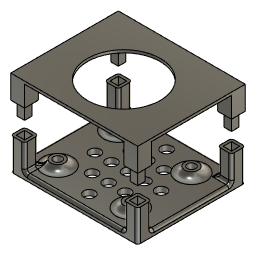
Joystick+Holder+Rev+3 (Autodesk Fusion 360 design; units mm, degrees)
Autodesk Fusion 360 part; units mm, degrees
sketch "Joystick Layout" plane through (0, 0, 0) normal (0, 0, 1) x (1, 0, 0)
  line L0 (15.6333, 7.2313) -> (49.6333, 7.2313)
  line L1 (49.6333, 7.2313) -> (49.6333, 34.2313)
  line L2 (49.6333, 34.2313) -> (15.6333, 34.2313)
  line L3 (15.6333, 34.2313) -> (15.6333, 7.2313)
  line L4 (23.1333, 10.7313) -> (39.1333, 10.7313)
  line L5 (39.1333, 10.7313) -> (39.1333, 26.7313)
  line L6 (39.1333, 26.7313) -> (23.1333, 26.7313)
  line L7 (23.1333, 26.7313) -> (23.1333, 10.7313)
  line L8 (26.1333, 10.7313) -> (36.1333, 10.7313)
  line L9 (36.1333, 10.7313) -> (36.1333, 8.2313)
  line L10 (36.1333, 8.2313) -> (26.1333, 8.2313)
  line L11 (26.1333, 8.2313) -> (26.1333, 10.7313)
  line L12 (23.1333, 13.7313) -> (20.6333, 13.7313)
  line L13 (20.6333, 13.7313) -> (20.6333, 23.7313)
  line L14 (20.6333, 23.7313) -> (23.1333, 23.7313)
  line L15 (23.1333, 23.7313) -> (23.1333, 13.7313)
  circle A0 centre (32.1333, 19.7313) radius 6
  circle A1 centre (32.1333, 19.7313) radius 2
  line L16 (30.681, 21.1063) -> (30.681, 18.3562)
  line L17 (33.681, 20.998) -> (33.681, 18.4645)
  circle A2 centre (18.1333, 9.7313) radius 1.5
  circle A3 centre (18.1333, 31.7313) radius 1.5
  circle A4 centre (44.6333, 31.7313) radius 1.5
  circle A5 centre (44.6333, 9.7313) radius 1.5
  circle A6 centre (32.1333, 19.7313) radius 13
  line L18 (9.6333, 40.2313) -> (55.6333, 40.2313)
  line L19 (55.6333, 40.2313) -> (55.6333, 1.2313)
  line L20 (55.6333, 1.2313) -> (9.6333, 1.2313)
  line L21 (9.6333, 1.2313) -> (9.6333, 40.2313)
  line L22 (9.6333, 40.2313) -> (14.6333, 40.2313)
  line L23 (14.6333, 40.2313) -> (14.6333, 35.2313)
  line L24 (14.6333, 35.2313) -> (9.6333, 35.2313)
  line L25 (9.6333, 35.2313) -> (9.6333, 40.2313)
  line L26 (55.6333, 40.2313) -> (50.6333, 40.2313)
  line L27 (50.6333, 40.2313) -> (50.6333, 35.2313)
  line L28 (50.6333, 35.2313) -> (55.6333, 35.2313)
  line L29 (55.6333, 35.2313) -> (55.6333, 40.2313)
  line L30 (9.6333, 1.2313) -> (14.6333, 1.2313)
  line L31 (14.6333, 1.2313) -> (14.6333, 6.2313)
  line L32 (14.6333, 6.2313) -> (9.6333, 6.2313)
  line L33 (9.6333, 6.2313) -> (9.6333, 1.2313)
  line L34 (55.6333, 1.2313) -> (50.6333, 1.2313)
  line L35 (50.6333, 1.2313) -> (50.6333, 6.2313)
  line L36 (50.6333, 6.2313) -> (55.6333, 6.2313)
  line L37 (55.6333, 6.2313) -> (55.6333, 1.2313)
  line L38 (10.6333, 39.2313) -> (13.6333, 39.2313)
  line L39 (13.6333, 39.2313) -> (13.6333, 36.2313)
  line L40 (13.6333, 36.2313) -> (10.6333, 36.2313)
  line L41 (10.6333, 36.2313) -> (10.6333, 39.2313)
  line L42 (51.6333, 39.2313) -> (54.6333, 39.2313)
  line L43 (54.6333, 39.2313) -> (54.6333, 36.2313)
  line L44 (54.6333, 36.2313) -> (51.6333, 36.2313)
  line L45 (51.6333, 36.2313) -> (51.6333, 39.2313)
  line L46 (51.6333, 5.2313) -> (54.6333, 5.2313)
  line L47 (54.6333, 5.2313) -> (54.6333, 2.2313)
  line L48 (54.6333, 2.2313) -> (51.6333, 2.2313)
  line L49 (51.6333, 2.2313) -> (51.6333, 5.2313)
  line L50 (10.6333, 5.2313) -> (13.6333, 5.2313)
  line L51 (13.6333, 5.2313) -> (13.6333, 2.2313)
  line L52 (13.6333, 2.2313) -> (10.6333, 2.2313)
  line L53 (10.6333, 2.2313) -> (10.6333, 5.2313)
  circle A7 centre (18.1333, 31.7313) radius 2.5
  circle A8 centre (44.6333, 31.7313) radius 2.5
  circle A9 centre (44.6333, 9.7313) radius 2.5
  circle A10 centre (18.1333, 9.7313) radius 2.5
  circle A11 centre (32.1333, 19.7313) radius 13.2
  line L54 (10.7833, 39.0813) -> (13.4833, 39.0813)
  line L55 (13.4833, 39.0813) -> (13.4833, 36.3813)
  line L56 (13.4833, 36.3813) -> (10.7833, 36.3813)
  line L57 (10.7833, 36.3813) -> (10.7833, 39.0813)
  line L58 (51.7833, 39.0813) -> (54.4833, 39.0813)
  line L59 (54.4833, 39.0813) -> (54.4833, 36.3813)
  line L60 (54.4833, 36.3813) -> (51.7833, 36.3813)
  line L61 (51.7833, 36.3813) -> (51.7833, 39.0813)
  line L62 (54.4833, 2.3813) -> (51.7833, 2.3813)
  line L63 (51.7833, 2.3813) -> (51.7833, 5.0813)
  line L64 (51.7833, 5.0813) -> (54.4833, 5.0813)
  line L65 (54.4833, 5.0813) -> (54.4833, 2.3813)
  line L66 (10.7833, 5.0813) -> (13.4833, 5.0813)
  line L67 (13.4833, 5.0813) -> (13.4833, 2.3813)
  line L68 (13.4833, 2.3813) -> (10.7833, 2.3813)
  line L69 (10.7833, 2.3813) -> (10.7833, 5.0813)
  dimension "d1" = 34
  dimension "d2" = 27
  dimension "d3" = 16
  dimension "d4" = 16
  dimension "d5" = 10
  dimension "d6" = 2.5
  dimension "d7" = 2.5
  dimension "d8" = 10
  dimension "d9" = 3
  dimension "d10" = 3
  dimension "d11" = 1
  dimension "d12" = 12
  dimension "d13" = 9
  dimension "d14" = 9
  dimension "d15" = 4
  dimension "d16" = 3
  dimension "d17" = 5
  dimension "d18" = 3
  dimension "d19" = 3
  dimension "d20" = 2.5
  dimension "d21" = 2.5
  dimension "d22" = 2.5
  dimension "d23" = 2.5
  dimension "d24" = 3
  dimension "d25" = 3
  dimension "d26" = 2.5
  dimension "d27" = 2.5
  dimension "d28" = 26.5
  dimension "d29" = 26.5
  dimension "d30" = 26
  dimension "d31" = 5
  dimension "d32" = 5
  dimension "d33" = 5
  dimension "d34" = 5
  dimension "d35" = 1
  dimension "d36" = 1
  dimension "d37" = 1
  dimension "d38" = 5
  dimension "d39" = 5
  dimension "d40" = 5
  dimension "d41" = 5
  dimension "d42" = 1
  dimension "d43" = 3
  dimension "d44" = 3
  dimension "d45" = 1
  dimension "d46" = 1
  dimension "d47" = 3
  dimension "d48" = 3
  dimension "d49" = 1
  dimension "d50" = 1
  dimension "d51" = 3
  dimension "d52" = 3
  dimension "d53" = 1
  dimension "d54" = 1
  dimension "d55" = 3
  dimension "d56" = 3
  dimension "d57" = 1
  dimension "d58" = 1
  dimension "d59" = 5
  dimension "d60" = 5
  dimension "d61" = 5
  dimension "d62" = 5
  dimension "d100" = 26.4
  dimension "d107" = 2.7
  dimension "d108" = 2.7
  dimension "d109" = 0.15
  dimension "d110" = 0.15
  dimension "d111" = 2.7
  dimension "d112" = 2.7
  dimension "d113" = 0.15
  dimension "d114" = 0.15
  dimension "d115" = 2.7
  dimension "d116" = 2.7
  dimension "d117" = 0.15
  dimension "d118" = 0.15
  dimension "d119" = 2.7
  dimension "d120" = 2.7
  dimension "d121" = 0.15
  dimension "d122" = 0.15
  constraint horizontal L0
  constraint vertical L1
  constraint horizontal L2
  constraint vertical L3
  constraint horizontal L4
  constraint vertical L5
  constraint horizontal L6
  constraint vertical L7
  constraint horizontal L8
  constraint vertical L9
  constraint horizontal L10
  constraint vertical L11
  constraint coincident L4 L8.start
  constraint horizontal L12
  constraint vertical L13
  constraint horizontal L14
  constraint vertical L15
  constraint coincident L7 L12.start
  constraint concentric A0 A1
  constraint coincident A1 L16.start
  constraint coincident A1 L16.end
  constraint vertical L16
  constraint coincident A1 L17.start
  constraint coincident A1 L17.end
  constraint parallel L16 L17
  constraint concentric A0 A6
  constraint horizontal L18
  constraint vertical L19
  constraint horizontal L20
  constraint vertical L21
  constraint horizontal L22
  constraint vertical L23
  constraint horizontal L24
  constraint vertical L25
  constraint horizontal L26
  constraint vertical L27
  constraint horizontal L28
  constraint vertical L29
  constraint horizontal L30
  constraint vertical L31
  constraint horizontal L32
  constraint vertical L33
  constraint horizontal L34
  constraint vertical L35
  constraint horizontal L36
  constraint vertical L37
  constraint horizontal L38
  constraint vertical L39
  constraint horizontal L40
  constraint vertical L41
  constraint horizontal L42
  constraint vertical L43
  constraint horizontal L44
  constraint vertical L45
  constraint horizontal L46
  constraint vertical L47
  constraint horizontal L48
  constraint vertical L49
  constraint horizontal L50
  constraint vertical L51
  constraint horizontal L52
  constraint vertical L53
  constraint concentric A3 A7
  constraint concentric A4 A8
  constraint concentric A5 A9
  constraint concentric A2 A10
  constraint concentric A1 A11
  constraint horizontal L54
  constraint vertical L55
  constraint horizontal L56
  constraint vertical L57
  constraint horizontal L58
  constraint vertical L59
  constraint horizontal L60
  constraint vertical L61
  constraint horizontal L62
  constraint vertical L63
  constraint horizontal L64
  constraint vertical L65
  constraint horizontal L66
  constraint vertical L67
  constraint horizontal L68
  constraint vertical L69
  measures "d1" distance of L0.start L0.end
  measures "d2" distance of L0.start L2.end
  measures "d3" distance of L4.start L4.end
  measures "d4" distance of L4.start L6.end
  measures "d5" distance of L8.start L8.end
  measures "d6" distance of L8.start L10.end
  measures "d7" distance of L12.start L12.end
  measures "d8" distance of L12.start L14.end
  measures "d9" distance of L4 L12
  measures "d10" distance of L7 L11
  measures "d11" distance of L0 L10
  measures "d12" diameter of A0
  measures "d13" distance of L8 A0.centre
  measures "d14" distance of L7 A0.centre
  measures "d15" diameter of A1
  measures "d16" distance of L16 L17
  measures "d17" distance of L3 L13
  measures "d18" diameter of A2
  measures "d19" diameter of A3
  measures "d20" distance of L3 A3.centre
  measures "d21" distance of L2 A3.centre
  measures "d22" distance of L3 A2.centre
  measures "d23" distance of L0 A2.centre
  measures "d24" diameter of A4
  measures "d25" diameter of A5
  measures "d26" distance of L0 A5.centre
  measures "d27" distance of L2 A4.centre
  measures "d28" distance of A3.centre A4.centre
  measures "d29" distance of A2.centre A5.centre
  measures "d30" diameter of A6
  measures "d31" distance of L18.start L22.end
  measures "d32" distance of L18.start L24.end
  measures "d33" distance of L18.end L26.end
  measures "d34" distance of L18.end L28.end
  measures "d35" distance of L3 L23
  measures "d36" distance of L2 L24
  measures "d37" distance of L1 L27
  measures "d38" distance of L20.end L30.end
  measures "d39" distance of L19.end L34.end
  measures "d40" distance of L19.end L36.end
  measures "d41" distance of L20.end L32.end
  measures "d42" distance of L0 L32
  measures "d43" distance of L38.start L38.end
  measures "d44" distance of L38.start L40.end
  measures "d45" distance of L18 L38
  measures "d46" distance of L25 L41
  measures "d47" distance of L42.start L42.end
  measures "d48" distance of L42.start L44.end
  measures "d49" distance of L19 L43
  measures "d50" distance of L18 L42
  measures "d51" distance of L46.start L46.end
  measures "d52" distance of L46.start L48.end
  measures "d53" distance of L36 L46
  measures "d54" distance of L37 L47
  measures "d55" distance of L50.start L50.end
  measures "d56" distance of L50.start L52.end
  measures "d57" distance of L32 L50
  measures "d58" distance of L31 L51
  measures "d59" diameter of A7
  measures "d60" diameter of A8
  measures "d61" diameter of A9
  measures "d62" diameter of A10
  measures "d100" diameter of A11
  measures "d107" distance of L54.start L54.end
  measures "d108" distance of L54.start L56.end
  measures "d109" distance of L38 L54
  measures "d110" distance of L41 L57
  measures "d111" distance of L58.start L58.end
  measures "d112" distance of L58.start L60.end
  measures "d113" distance of L42 L58
  measures "d114" distance of L45 L61
  measures "d115" distance of L62.start L62.end
  measures "d116" distance of L62.start L64.end
  measures "d117" distance of L46 L64
  measures "d118" distance of L49 L63
  measures "d119" distance of L66.start L66.end
  measures "d120" distance of L66.start L68.end
  measures "d121" distance of L50 L66
  measures "d122" distance of L53 L69
extrude "Extrude1" add sketch "Joystick Layout" along normal blind 1 contours L0 L3 A10 | L0 L1 L2 L3 A7 A10 A11 | L0 A6 A11 | L0 A6 A11 | L2 L3 A7 | L0 A6 | L0 A6 | L4 L5 L6 L7 L8 L15 | L4 L8 L9 L10 L11 | L7 L12 L13 L14 L15 | A0 | A1 L17 | A1 L16 L17 | A1 L16 | L18 L19 L20 L21 L23 L24 L27 L28 L31 L32 L35 L36 makes body 1
extrude "Extrude2" add sketch "Joystick Layout" along normal blind 3 contours A9 | A8 | A10 | A7 bodies 1
extrude "Extrude3" add sketch "Joystick Layout" along normal blind 10.5 contours L18 L21 L22 L23 L24 L25 | L18 L19 L26 L27 L28 L29 | L20 L21 L30 L31 L32 L33 | L19 L20 L34 L35 L36 L37 bodies 1
extrude "Extrude4" add sketch "Joystick Layout" along normal blind 3 contours L38 L39 L40 L41 | L42 L43 L44 L45 | L46 L47 L48 L49 | L50 L51 L52 L53 | L54 L55 L56 L57 | L58 L59 L60 L61 | L62 L63 L64 L65 | L66 L67 L68 L69 bodies 1
fillet "Fillet1" radius 3 4 edges at (42.3025, 32.6353, 1) (42.3025, 10.6353, 1) (15.8025, 10.6353, 1) (15.8025, 32.6353, 1) on bodies 1
fillet "Fillet2" radius 1 12 edges at (53.1333, 6.2313, 1) (50.6333, 3.7313, 1) (11.8745, 6.2313, 1) (14.3692, 6.2313, 1.006) (14.6333, 5.9671, 1.006) (14.6333, 3.4724, 1) (53.1333, 35.2313, 1) (50.6333, 37.7313, 1) (14.3692, 35.2313, 1.006) (11.8745, 35.2313, 1) (14.6333, 37.9901, 1) (14.6333, 35.4954, 1.006) on bodies 1
fillet "Fillet3" radius 1 2 edges at (15.3836, 6.9815, 1.5924) (14.6333, 6.2313, 6.392) on bodies 1
fillet "Fillet4" radius 1 5 edges at (50.6333, 1.2313, 6.25) (50.3404, 1.2313, 1.2929) (32.6333, 1.2313, 1) (14.9262, 1.2313, 1.2929) (14.6333, 1.2313, 6.25) on bodies 1
fillet "Fillet5" radius 1 19 edges at (9.6333, 1.2313, 5.25) (9.6333, 35.2313, 6.25) (9.6333, 34.9384, 1.2929) (9.6333, 20.7313, 1) (9.6333, 6.5241, 1.2929) (9.6333, 6.2313, 6.25) (9.6333, 40.2313, 5.25) (50.6333, 40.2313, 6.25) (50.3404, 40.2313, 1.2929) (32.6333, 40.2313, 1) (14.9262, 40.2313, 1.2929) (14.6333, 40.2313, 6.25) (55.6333, 40.2313, 5.25) (55.6333, 6.2313, 6.25) (55.6333, 6.5241, 1.2929) (55.6333, 20.7313, 1) (55.6333, 34.9384, 1.2929) (55.6333, 35.2313, 6.25) (55.6333, 1.2313, 5.25) on bodies 1
fillet "Fillet6" radius 1 6 edges at (50.3404, 34.9384, 1.2929) (50.6333, 35.2313, 6.25) (15.3836, 34.481, 1.5924) (14.6333, 35.2313, 6.392) (50.3404, 6.5241, 1.2929) (50.6333, 6.2313, 6.25) on bodies 1
extrude "Extrude5" add 1 faces at (27.3332, 24.0578, 0) along direction (0, 0, -1) blind 1 on bodies 1 bodies 1
sketch "Holes" plane through (0, 0, 1) normal (0, 0, 1) x (-1, 0, 0)
  circle A0 centre (-44.6333, -9.7313) radius 5.3284
  circle A1 centre (-44.6333, -31.7313) radius 5.3284
  line L0 (-54.6333, -7.2313) -> (-54.6333, -34.2313)
  line L1 (-54.6333, -34.2313) -> (-49.6333, -34.2313)
  line L2 (-49.6333, -34.2313) -> (-49.6333, -39.2313)
  line L3 (-49.6333, -39.2313) -> (-15.6333, -39.2313)
  line L4 (-15.6333, -39.2313) -> (-15.6333, -36.4368)
  arc A2 (-13.4278, -34.2313) -> (-15.6333, -36.4368) centre (-18.1333, -31.7313) ccw
  line L5 (-13.4278, -34.2313) -> (-10.6333, -34.2313)
  line L6 (-10.6333, -34.2313) -> (-10.6333, -7.2313)
  line L7 (-10.6333, -7.2313) -> (-13.4278, -7.2313)
  arc A3 (-15.6333, -5.0257) -> (-13.4278, -7.2313) centre (-18.1333, -9.7313) ccw
  line L8 (-15.6333, -5.0257) -> (-15.6333, -2.2313)
  line L9 (-15.6333, -2.2313) -> (-49.6333, -2.2313)
  line L10 (-49.6333, -2.2313) -> (-49.6333, -7.2313)
  line L11 (-49.6333, -7.2313) -> (-54.6333, -7.2313)
  circle A4 centre (-32.8333, -20.5313) radius 2
  circle A5 centre (-26.8333, -20.5313) radius 2
  circle A6 centre (-20.8333, -20.5313) radius 2
  circle A7 centre (-14.8333, -20.5313) radius 2
  circle A8 centre (-32.8333, -13.5313) radius 2
  circle A9 centre (-26.8333, -13.5313) radius 2
  circle A10 centre (-20.8333, -13.5313) radius 2
  circle A11 centre (-14.8333, -13.5313) radius 2
  circle A12 centre (-32.8333, -6.5313) radius 2
  circle A13 centre (-26.8333, -6.5313) radius 2
  circle A14 centre (-20.8333, -6.5313) radius 2
  circle A15 centre (-14.8333, -6.5313) radius 2
  circle A16 centre (-38.8333, -20.5313) radius 2
  circle A17 centre (-44.8333, -20.5313) radius 2
  circle A18 centre (-50.8333, -20.5313) radius 2
  circle A19 centre (-32.8333, -13.5313) radius 2
  circle A20 centre (-38.8333, -13.5313) radius 2
  circle A21 centre (-44.8333, -13.5313) radius 2
  circle A22 centre (-50.8333, -13.5313) radius 2
  circle A23 centre (-32.8333, -6.5313) radius 2
  circle A24 centre (-38.8333, -6.5313) radius 2
  circle A25 centre (-44.8333, -6.5313) radius 2
  circle A26 centre (-50.8333, -6.5313) radius 2
  circle A27 centre (-14.8333, -27.5313) radius 2
  circle A28 centre (-20.8333, -27.5313) radius 2
  circle A29 centre (-26.8333, -27.5313) radius 2
  circle A30 centre (-32.8333, -27.5313) radius 2
  circle A31 centre (-38.8333, -27.5313) radius 2
  circle A32 centre (-44.8333, -27.5313) radius 2
  circle A33 centre (-50.8333, -27.5313) radius 2
  circle A34 centre (-14.8333, -34.5313) radius 2
  circle A35 centre (-20.8333, -34.5313) radius 2
  circle A36 centre (-26.8333, -34.5313) radius 2
  circle A37 centre (-32.8333, -34.5313) radius 2
  circle A38 centre (-38.8333, -34.5313) radius 2
  circle A39 centre (-44.8333, -34.5313) radius 2
  circle A40 centre (-50.8333, -34.5313) radius 2
  dimension "d85" = 4
  dimension "d88" = 18
  dimension "d89" = 14
  dimension "d92" = -18
  dimension "d93" = 14
  dimension "d96" = 0
  dimension "d97" = -14
  measures "d85" diameter of A4
extrude "Extrude6" cut sketch "Holes" against normal blind 2 contours A0 A20 | A1 A31 | A4 | A5 | A6 | A8 A19 | A9 | A12 A23 | A16 | A17 | A29 | A30 | A37 picked at (-39.1764, -13.3043) picked at (-39.2731, -27.8765) bodies 1
extrude "Extrude13" add sketch "Joystick Layout" along normal blind 1 separate body contours L0 L3 A10 | A9 | A8 | L0 L1 L2 L3 A7 A10 A11 | A10 | L2 L3 A7 | A7 | A2 | A3 | A4 | A5 | L18 L21 L22 L23 L24 L25 | L18 L19 L20 L21 L23 L24 L27 L28 L31 L32 L35 L36 | L18 L19 L26 L27 L28 L29 | L20 L21 L30 L31 L32 L33 | L19 L20 L34 L35 L36 L37 | L38 L39 L40 L41 | L42 L43 L44 L45 | L46 L47 L48 L49 | L50 L51 L52 L53 | L54 L55 L56 L57 | L58 L59 L60 L61 | L62 L63 L64 L65 | L66 L67 L68 L69 makes body 2
extrude "Extrude16" add sketch "Joystick Layout" against normal blind 7.5 contours L18 L21 L22 L23 L24 L25 | L18 L19 L26 L27 L28 L29 | L20 L21 L30 L31 L32 L33 | L19 L20 L34 L35 L36 L37 | L38 L39 L40 L41 | L42 L43 L44 L45 | L46 L47 L48 L49 | L50 L51 L52 L53 bodies 2
extrude "Extrude17" add 4 faces at (11.6833, 38.1813, 0) (11.6833, 4.1813, 0) (52.6833, 4.1813, 0) (52.6833, 38.1813, 0) along direction (0, 0, -1) blind 12.5 on bodies 2 bodies 2
copy_body "Body->Comp1" bodies 1 removing the originals makes body 3 in component "Bottom"
copy_body "Body->Comp2" bodies 2 removing the originals makes body 4 in component "Face"
component "Bottom" placed x (1, 0, 0) y (0, 1, 0) z (0, 0, 1) at (0, 0, 0)
component "Face" placed x (1, 0, 0) y (0, 1, 0) z (0, 0, 1) at (0, 0, 0)
equation "d137 = 7.5 mm + 5 mm"
named bodies: "Bottom", "Face"
